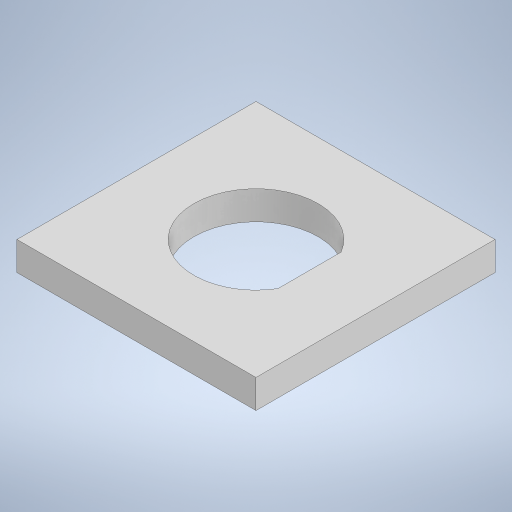
# Autodesk Inventor part: StartBtnMount_test
Saved by Autodesk Inventor 2024.2 (Build 282272000, 272)
## iProperties
Created: 2024-04-16
Part Number: StartBtnMount_test
Material: Generic
Document SubType Name: Modeling
Designer: ringl
Density: 1 g/cm^3
Appearance: Default
Author: ringl
Autodesk Inventor part; units mm, degrees
ref_plane "YZ Plane" through (0, 0, 0) normal (1, 0, 0) x (0, 1, 0)
ref_plane "XZ Plane" through (0, 0, 0) normal (0, 1, 0) x (-1, 0, 0)
ref_plane "XY Plane" through (0, 0, 0) normal (0, 0, 1) x (1, 0, 0)
sketch "Sketch1" plane through (0, 0, 0) normal (0, 1, 0) x (-1, 0, 0)
  line L0 (0, 0) -> (25, 0)
  line L1 (25, 0) -> (25, -25)
  line L2 (25, -25) -> (0, -25)
  line L3 (0, -25) -> (0, 0)
  arc A0 (6.9, -15.8) -> (6.9, -9.2) centre (12.5, -12.5) ccw
  line L4 (6.9, -15.8) -> (6.9, -9.2)
  point P0 (25, -12.5)
  dimension "d0" = 13
  dimension "d1" = 25
  dimension "d2" = 25
  dimension "d3" = 12.5
  dimension "d4" = 12.5
  dimension "d7" = 5.6
  constraints: 10 end point, 2 parallel, 2 point on circle, 1 centre point, 1 horizontal, 1 midpoint, 1 perpendicular, 1 vertical
  measures "d0" diameter of A0
  measures "d1" distance of L1.end L2.end
  measures "d2" distance of L0.end L1.end
  measures "d3" distance from line of L0 A0.centre
  measures "d4" distance of point (25, -12.5) A0.centre
  measures "d7" distance from line of A0.centre L4
extrude "Extrusion1" add sketch "Sketch1" along normal blind 3
body "Solid1"
